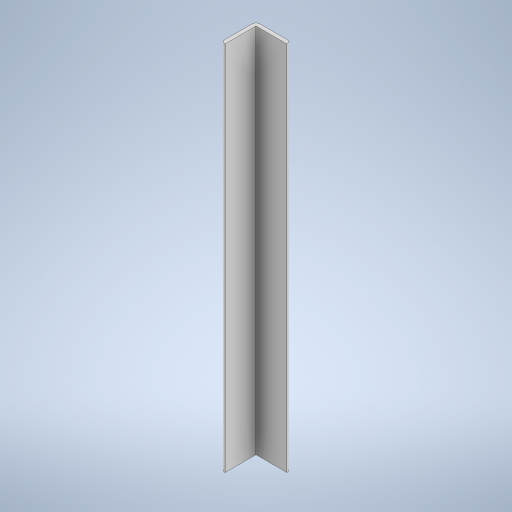
# Autodesk Inventor part: Cargo Aluminum L
Saved by Autodesk Inventor 2024.2 (Build 282272000, 272)
## iProperties
Created: 2023-11-13
Part Number: Cargo Aluminum L
Material: Generic
Document SubType Name: Modeling
Designer: Luke
Density: 1 g/cm^3
Appearance: Default
Author: Luke
Autodesk Inventor part; units mm, degrees
ref_plane "YZ Plane" through (0, 0, 0) normal (1, 0, 0) x (0, 1, 0)
ref_plane "XZ Plane" through (0, 0, 0) normal (0, 1, 0) x (-1, 0, 0)
ref_plane "XY Plane" through (0, 0, 0) normal (0, 0, 1) x (1, 0, 0)
sketch "Sketch1" plane through (0, 0, 0) normal (0, 1, 0) x (-1, 0, 0)
  line L0 (22.344, 28.575) -> (19.169, 28.575)
  line L1 (19.169, 28.575) -> (19.169, 0)
  line L2 (19.169, 0) -> (22.344, 0)
  line L3 (22.344, 0) -> (22.344, 28.575)
  line L4 (22.344, 0) -> (-6.231, 0)
  line L5 (-6.231, 0) -> (-6.231, 3.175)
  line L6 (-6.231, 3.175) -> (22.344, 3.175)
  line L7 (22.344, 3.175) -> (22.344, 0)
  point P0 (0, 0)
  point P1 (20.7565, 0)
  point P2 (20.7565, 28.575)
  point P3 (19.169, 3.175)
  point P4 (19.169, 0)
  dimension "d0" = 3.175
  dimension "d1" = 3.175
  dimension "d2" = 28.575
  dimension "d3" = 28.575
  constraints: 16 end point, 4 parallel, 2 horizontal, 2 midpoint, 2 perpendicular
  measures "d0" distance of L2.end L1.end
  measures "d1" distance between parallel lines of L4 L6
  measures "d2" distance of L2.end L4.end
  measures "d3" distance of point (20.756, 0) point (20.756, 28.575)
extrude "Extrusion1" add sketch "Sketch1" along normal blind 304.8
fillet "Fillet1" radius 3.175 3 edges at (6.231, 152.4, 0) (-22.344, 152.4, 0) (-22.344, 152.4, 28.575)
body "Solid1"
